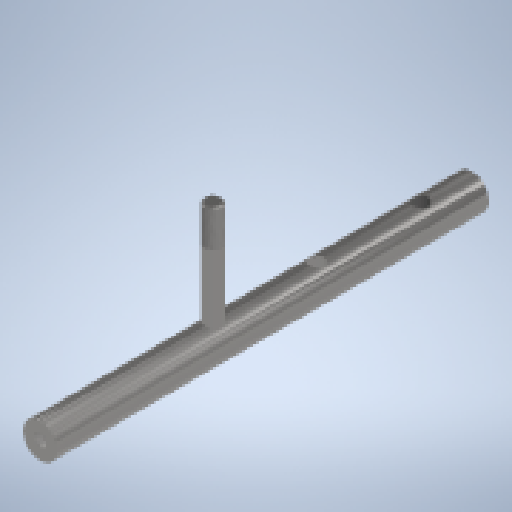
# Autodesk Inventor part: Ruderstange
Saved by Autodesk Inventor 2024.4 (Build 284460000, 460)
## iProperties
Created: 2026-01-12
Part Number: Ruderstange
Material: Edelstahl
Document SubType Name: Modeling
Designer: PC
Density: 8 g/cm^3
Appearance: Halbpoliert
Description: Ruderstange
Mass: 641.963 g
Surface Area: 194.722 cm^2
Volume: 80.2453 cm^3
Masse[kg]: 0,558 kg
Autodesk Inventor part; units mm, degrees
ref_plane "YZ Plane" through (0, 0, 0) normal (1, 0, 0) x (0, 1, 0)
ref_plane "XZ Plane" through (0, 0, 0) normal (0, 1, 0) x (-1, 0, 0)
sketch "Skizze1" plane through (0, 0, 0) normal (0, 1, 0) x (-1, 0, 0)
  circle A0 centre (0, 0) radius 10
  dimension "d17" = 20
  constraints: 1 centre point
  measures "d17" diameter of A0
extrude "Extrusion1" add sketch "Skizze1" along normal blind 250
sketch "Skizze4" plane through (0, 0, 0) normal (0, 0, 1) x (1, 0, 0)
  line L0 (0, 0) -> (0, 100)
  circle A0 centre (0, 100) radius 5
  dimension "d10" = 100
  dimension "d11" = 10
  constraints: 2 end point, 1 centre point, 1 coincident, 1 vertical
  measures "d10" distance of L0.start L0.end
  measures "d11" diameter of A0
extrude "Extrusion3" add sketch "Skizze4" along normal blind 70
ref_plane "Arbeitsebene1" through (0, 0, 3.5) normal (0, 0, 1) x (1, 0, 0)
sketch "Skizze6" plane through (0, 0, 3.5) normal (0, 0, 1) x (1, 0, 0)
  line L0 (10, 250) -> (-10, 250) projected
  line L1 (0, 250) -> (0, 220)
  circle A0 centre (0, 220) radius 4.25
  line L2 (0, 220) -> (0, 160)
  circle A1 centre (0, 160) radius 4.25
  point P0 (0, 0)
  dimension "d19" = 30
  dimension "d20" = 8.5
  dimension "d21" = 60
  dimension "d22" = 8.5
  constraints: 4 end point, 2 centre point, 2 coincident, 2 vertical, 1 midpoint
  measures "d19" distance of L1.start L1.end
  measures "d20" diameter of A0
  measures "d21" distance of L2.start L2.end
  measures "d22" diameter of A1
extrude "Extrusion5" cut sketch "Skizze6" along normal through all both and the other way through all
chamfer "Fasen1" distance 1 angle 45 1 edges at (-5, 100, 70)
thread "Gewinde2" size "M10x1.5" class "6g" standard "ANSI Metric M Profile" length 20
sketch "Skizze7" plane through (0, 0, 0) normal (0, -1, 0) x (1, 0, 0)
  point P0 (0, 0)
hole "Bohrung1" at (0, 0, 0) direction (0, 1, 0) diameter 6.647 depth 22.2 tip angle 118 thread size "M8x1.25" class "6H" standard "ISO Metric profile"
